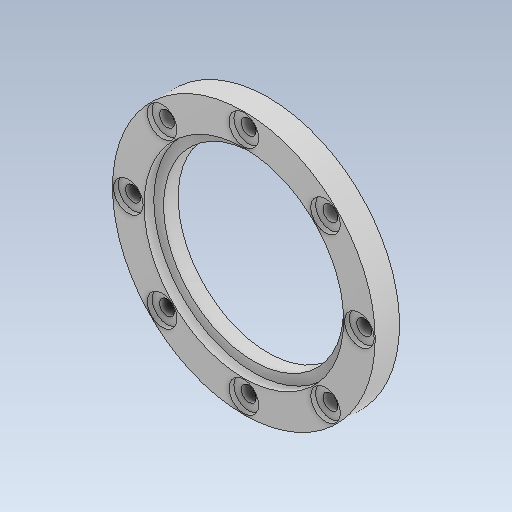
# Autodesk Inventor part: Outer_support_stand
Saved by Autodesk Inventor 2020.4 (Build 244396000, 396)
## iProperties
Created: 2021-09-25
Part Number: Outer_support_stand
Material: アルミニウム 2014-T4
Document SubType Name: Modeling
Designer: Masato
Density: 2.8 g/cm^3
Appearance: 滑らか - 淡い灰色
Author: Masato
Autodesk Inventor part; units mm, degrees
ref_plane "YZ Plane" through (0, 0, 0) normal (1, 0, 0) x (0, 1, 0)
ref_plane "XZ Plane" through (0, 0, 0) normal (0, 1, 0) x (-1, 0, 0)
ref_plane "XY Plane" through (0, 0, 0) normal (0, 0, 1) x (1, 0, 0)
derived "Trunk_horizontal_frame_01.ipt"
sketch "スケッチ1" plane through (0, 0, 0) normal (0, 0, 1) x (1, 0, 0)
  line L0 (-62, 30.75) -> (62, 30.75)
  line L1 (62, -30.75) -> (-62, -30.75)
  line L2 (-62, 30.75) -> (62, -30.75) construction
  line L3 (62, 30.75) -> (-62, -30.75) construction
  line L4 (0, 30.75) -> (0, -30.75) construction
  circle A0 centre (-44, 2.25) radius 10.5 construction
  line L5 (-57.5, 1.25) -> (-30.5, 1.25) construction
  line L6 (-30.5, 1.25) -> (-30.5, -25.75) construction
  line L7 (-30.5, -25.75) -> (-57.5, -25.75) construction
  line L8 (-57.5, -25.75) -> (-57.5, 1.25) construction
  line L9 (-44, 1.25) -> (-44, -25.75) construction
  line L10 (-57.5, -12.25) -> (-30.5, -12.25) construction
  circle A1 centre (-57.5, 1.25) radius 1.35
  circle A2 centre (-57.5, -25.75) radius 1.35
  circle A3 centre (-30.5, 1.25) radius 1.35
  circle A4 centre (-30.5, -25.75) radius 1.35
  line L11 (-27.5, 21.75) -> (-22.5, 21.75) construction
  line L12 (-22.5, 21.75) -> (-22.5, 11.75) construction
  line L13 (-22.5, 11.75) -> (-27.5, 11.75) construction
  line L14 (-27.5, 11.75) -> (-27.5, 21.75) construction
  line L15 (-27.5, 21.75) -> (-22.5, 11.75) construction
  line L16 (-22.5, 21.75) -> (-27.5, 11.75) construction
  line L17 (-27.51, 21.76) -> (-22.49, 21.76)
  line L18 (-22.49, 21.76) -> (-22.49, 11.74)
  line L19 (-22.49, 11.74) -> (-27.51, 11.74)
  line L20 (-27.51, 11.74) -> (-27.51, 21.76)
  line L21 (-27.51, 21.76) -> (-22.49, 11.74) construction
  line L22 (-22.49, 21.76) -> (-27.51, 11.74) construction
  line L23 (-27.51, 16.75) -> (-22.49, 16.75) construction
  line L24 (-25, 21.76) -> (-25, 11.74) construction
  arc A5 (-27.51, 21.76) -> (-27.51, 19.66) centre (-27.51, 20.71) ccw
  arc A6 (-22.49, 19.66) -> (-22.49, 21.76) centre (-22.49, 20.71) ccw
  arc A7 (-22.49, 11.74) -> (-22.49, 13.84) centre (-22.49, 12.79) ccw
  arc A8 (-27.51, 13.84) -> (-27.51, 11.74) centre (-27.51, 12.79) ccw
  circle A9 centre (-25, 27.75) radius 1.55
  arc A10 (-27.51, -19.66) -> (-27.51, -21.76) centre (-27.51, -20.71) ccw
  line L25 (-22.5, -21.75) -> (-27.5, -21.75) construction
  line L26 (-22.49, -21.76) -> (-27.51, -21.76)
  arc A11 (-22.49, -21.76) -> (-22.49, -19.66) centre (-22.49, -20.71) ccw
  line L27 (-27.5, -21.75) -> (-27.5, -9.25) construction
  line L28 (-27.51, -21.76) -> (-27.51, -9.24)
  line L29 (-27.51, -15.5) -> (-22.49, -15.5) construction
  line L30 (-25, -9.24) -> (-25, -21.76) construction
  line L31 (-27.5, -9.25) -> (-22.5, -21.75) construction
  line L32 (-22.5, -9.25) -> (-27.5, -21.75) construction
  line L33 (-27.51, -9.24) -> (-22.49, -21.76) construction
  line L34 (-22.49, -9.24) -> (-27.51, -21.76) construction
  line L35 (-22.5, -9.25) -> (-22.5, -21.75) construction
  line L36 (-22.49, -9.24) -> (-22.49, -21.76)
  circle A12 centre (-25, -27.75) radius 1.55
  arc A13 (-22.49, -11.34) -> (-22.49, -9.24) centre (-22.49, -10.29) ccw
  line L37 (-27.5, -9.25) -> (-22.5, -9.25) construction
  line L38 (-27.51, -9.24) -> (-22.49, -9.24)
  arc A14 (-27.51, -9.24) -> (-27.51, -11.34) centre (-27.51, -10.29) ccw
  circle A15 centre (-44, 2.25) radius 11
  line L39 (62, 2.25) -> (-62, 2.25) construction
  line L40 (-60, 14.25) -> (-28, 14.25) construction
  line L41 (-28, 14.25) -> (-28, -28.75) construction
  line L42 (-28, -28.75) -> (-60, -28.75) construction
  line L43 (-60, -28.75) -> (-60, 14.25) construction
  line L44 (-60, 14.25) -> (-28, -28.75) construction
  line L45 (-28, 14.25) -> (-60, -28.75) construction
  line L46 (-62, 30.75) -> (-62, -30.75) construction
  line L47 (62, 30.75) -> (62, -30.75) construction
  circle A16 centre (-44, 2.25) radius 12.5 construction
  circle A17 centre (-44, 2.25) radius 20.5 construction
  circle A18 centre (-44, 2.25) radius 27 construction
  circle A19 centre (-44, 2.25) radius 28.75 construction
  circle A20 centre (-44, 26) radius 2.2 construction
  circle A21 centre (-60.7938, 19.0438) radius 2.2 construction
  circle A22 centre (-67.75, 2.25) radius 2.2 construction
  circle A23 centre (-60.7938, -14.5438) radius 2.2 construction
  circle A24 centre (-44, -21.5) radius 2.2 construction
  circle A25 centre (-27.2062, -14.5438) radius 2.2 construction
  circle A26 centre (-20.25, 2.25) radius 2.2 construction
  circle A27 centre (-27.2062, 19.0438) radius 2.2 construction
  arc A28 (-40.2168, 30.75) -> (-62, -20.1679) centre (-44, 2.25) ccw
  line L48 (-62, -20.1679) -> (-62, -30.75)
  arc A29 (22.49, -9.24) -> (22.49, -11.34) centre (22.49, -10.29) ccw
  line L49 (27.51, -9.24) -> (22.49, -9.24)
  arc A30 (27.51, -11.34) -> (27.51, -9.24) centre (27.51, -10.29) ccw
  line L50 (27.51, -21.76) -> (27.51, -9.24)
  line L51 (22.49, -9.24) -> (22.49, -21.76)
  circle A31 centre (27.2062, -14.5438) radius 2.2
  arc A32 (27.51, -21.76) -> (27.51, -19.66) centre (27.51, -20.71) ccw
  line L52 (22.49, -21.76) -> (27.51, -21.76)
  arc A33 (22.49, -19.66) -> (22.49, -21.76) centre (22.49, -20.71) ccw
  circle A34 centre (25, -27.75) radius 1.55
  circle A35 centre (30.5, -25.75) radius 1.35
  circle A36 centre (44, -21.5) radius 2.2
  circle A37 centre (57.5, -25.75) radius 1.35
  circle A38 centre (60.7938, -14.5438) radius 2.2
  line L53 (62, -20.1679) -> (62, -30.75)
  circle A39 centre (67.75, 2.25) radius 2.2
  circle A40 centre (60.7938, 19.0438) radius 2.2
  circle A41 centre (44, 26) radius 2.2
  circle A42 centre (44, 2.25) radius 11
  circle A43 centre (27.2062, 19.0438) radius 2.2
  circle A44 centre (25, 27.75) radius 1.55
  circle A45 centre (30.5, 1.25) radius 1.35
  circle A46 centre (57.5, 1.25) radius 1.35
  circle A47 centre (20.25, 2.25) radius 2.2
  line L54 (22.49, 11.74) -> (27.51, 11.74)
  arc A48 (27.51, 11.74) -> (27.51, 13.84) centre (27.51, 12.79) ccw
  arc A49 (22.49, 13.84) -> (22.49, 11.74) centre (22.49, 12.79) ccw
  line L55 (22.49, 21.76) -> (22.49, 11.74)
  line L56 (27.51, 11.74) -> (27.51, 21.76)
  arc A50 (22.49, 21.76) -> (22.49, 19.66) centre (22.49, 20.71) ccw
  line L57 (27.51, 21.76) -> (22.49, 21.76)
  arc A51 (27.51, 19.66) -> (27.51, 21.76) centre (27.51, 20.71) ccw
  arc A52 (62, -20.1679) -> (40.2168, 30.75) centre (44, 2.25) ccw
  circle A53 centre (-44, 2.25) radius 20.51
  circle A54 centre (-44, 2.25) radius 18.5
  circle A55 centre (-44, 2.25) radius 27
  circle A56 centre (-44, 26) radius 1.55
  circle A57 centre (-60.7938, 19.0438) radius 1.55
  circle A58 centre (-67.75, 2.25) radius 1.55
  circle A59 centre (-60.7938, -14.5438) radius 1.55
  circle A60 centre (-44, -21.5) radius 1.55
  circle A61 centre (-27.2062, -14.5438) radius 1.55
  circle A62 centre (-20.25, 2.25) radius 1.55
  circle A63 centre (-27.2062, 19.0438) radius 1.55
  line L58 (-67.75, 2.25) -> (-72.75, 2.25) construction
  circle A64 centre (-27.2062, 19.0438) radius 7.2 construction
  circle A65 centre (-20.25, 2.25) radius 7.2 construction
  circle A66 centre (-27.2062, -14.5438) radius 7.2 construction
  circle A67 centre (-44, 2.25) radius 23.75 construction
  circle A68 centre (-44, 26) radius 3.05
  circle A69 centre (-60.7938, 19.0438) radius 3.05
  circle A70 centre (-67.75, 2.25) radius 3.05
  circle A71 centre (-44, -21.5) radius 3.05
  circle A72 centre (-27.2062, -14.5438) radius 3.05
  circle A73 centre (-20.25, 2.25) radius 3.05
  circle A74 centre (-27.2062, 19.0438) radius 3.05
  circle A75 centre (-60.7938, -14.5438) radius 3.05
  point P0 (0, 0)
  point P1 (-25, 16.75)
  point P2 (-25, -15.5)
  point P3 (-44, -7.25)
  dimension "d2" = 0.01
  dimension "d3" = 37
  dimension "d4" = 3.1
  dimension "d5" = 3.1
  dimension "d6" = 3.1
  dimension "d7" = 3.1
  dimension "d8" = 3.1
  dimension "d9" = 3.1
  dimension "d10" = 3.1
  dimension "d11" = 3.1
  dimension "d16" = 6.1
  dimension "d17" = 6.1
  dimension "d18" = 6.1
  dimension "d20" = 6.1
  dimension "d21" = 6.1
  dimension "d22" = 6.1
  dimension "d23" = 6.1
  dimension "d24" = 6.1
  measures "d2" radial gap between concentric circles of A17 A53
  measures "d3" diameter of A54
  measures "d4" diameter of A56
  measures "d5" diameter of A57
  measures "d6" diameter of A58
  measures "d7" diameter of A59
  measures "d8" diameter of A60
  measures "d9" diameter of A61
  measures "d10" diameter of A62
  measures "d11" diameter of A63
  measures "d16" diameter of A68
  measures "d17" diameter of A69
  measures "d18" diameter of A70
  measures "d20" diameter of A71
  measures "d21" diameter of A72
  measures "d22" diameter of A73
  measures "d23" diameter of A74
  measures "d24" diameter of A75
extrude "押し出し1" add sketch "スケッチ1" along normal blind 5 contours A74 L20 A53 A14 L28 A72 A55 L17 | L17 A55 L18 L19 A53 L20 A74 | A55 L36 A13 L38 A53 L19 A7 L18 | L28 A72 A53 L38 L36 A55 | A7 L18 | A53 L28 A14 | L36 A13 picked at (-27.7734, -10.754)
extrude "押し出し2" add sketch "スケッチ1" along normal blind 3 contours A53 L19 L20 | L20 A8 L19 A53 L38 A14 | L20 A8 | A14 L28 A53 | L38 A53 L28 picked at (-27.8728, -9.9602)
extrude "押し出し3" add sketch "スケッチ1" along normal blind 4 contours A5 A63 L20 A74 L17 | L17 A74 L20 A63 | L20 A63 A5 | A72 L28 A61 | L28 A61 A72 | A68 | A69 | A70 | A71 | A73 | A75 picked at (-27.8494, 20.8392)
equation "\"d5\" = d4"
equation "\"d6\" = d4"
equation "\"d7\" = d4"
equation "\"d8\" = d4"
equation "\"d9\" = d4"
equation "\"d10\" = d4"
equation "\"d11\" = d4"
equation "\"d17\" = d16"
equation "\"d18\" = d16"
equation "\"d20\" = d16"
equation "\"d21\" = d16"
equation "\"d22\" = d16"
equation "\"d23\" = d16"
equation "\"d24\" = d16"
